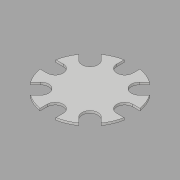
# Autodesk Inventor part: turntable
Saved by Autodesk Inventor 2017 (Build 210142000, 142)
## iProperties
Created: 2019-05-09
Part Number: turntable
Material: Generic
Document SubType Name: Modeling
Designer: Joe Sedutto
Density: 1 g/cm^3
Appearance: Default
Author: Joe Sedutto
Autodesk Inventor part; units mm, degrees
ref_plane "YZ Plane" through (0, 0, 0) normal (1, 0, 0) x (0, 1, 0)
ref_plane "XZ Plane" through (0, 0, 0) normal (0, 1, 0) x (-1, 0, 0)
ref_plane "XY Plane" through (0, 0, 0) normal (0, 0, 1) x (1, 0, 0)
sketch "Sketch1" plane through (0, 0, 0) normal (0, 1, 0) x (-1, 0, 0)
  circle A0 centre (0, 0) radius 34.925
  line L0 (0, 0) -> (0, -152.4) construction
  circle A1 centre (-107.7631, -44.6369) radius 34.925
  circle A2 centre (-152.4, -152.4) radius 34.925
  circle A3 centre (-107.7631, -260.1631) radius 34.925
  circle A4 centre (0, -304.8) radius 34.925
  circle A5 centre (107.7631, -260.1631) radius 34.925
  circle A6 centre (152.4, -152.4) radius 34.925
  circle A7 centre (107.7631, -44.6369) radius 34.925
  circle A8 centre (0, -152.4) radius 187.325
  dimension "d0" = 69.85
  dimension "d1" = 152.4
  dimension "d4" = 360
  constraints: 9 centre point, 2 coincident, 2 end point, 1 tangent, 1 vertical, 17 other
  measures "d0" diameter of A0
  measures "d1" distance of L0.end point (0, 0)
extrude "Extrusion1" add sketch "Sketch1" along normal blind 10
sketch "Sketch2" plane through (107.7631, 10, -44.6369) normal (0, 1, 0) x (1, 0, 0)
  arc A0 (-142.6881, -44.6369) -> (-72.8381, -44.6369) centre (-107.7631, -44.6369) ccw
  arc A1 (-142.6881, -76.2774) -> (-72.8381, -76.2774) centre (-107.7631, 107.7631) ccw
  line L0 (-72.8381, -44.6369) -> (-72.8381, -76.2774)
  line L1 (-142.6881, -44.6369) -> (-142.6881, -76.2774)
  circle A2 centre (-107.7631, -44.6369) radius 34.925 projected
  arc A3 (79.5619, 107.7631) -> (24.6957, 240.2219) centre (-107.7631, 107.7631) ccw projected
  arc A4 (-24.6957, -24.6957) -> (24.6957, 24.6957) centre (0, 0) ccw
  arc A5 (-2.3225, -47.0689) -> (47.0689, 2.3225) centre (-107.7631, 107.7631) ccw
  line L2 (24.6957, 24.6957) -> (47.0689, 2.3225)
  line L3 (-24.6957, -24.6957) -> (-2.3225, -47.0689)
  arc A6 (44.6369, 72.8381) -> (44.6369, 142.6881) centre (44.6369, 107.7631) ccw
  arc A7 (76.2774, 72.8381) -> (76.2774, 142.6881) centre (-107.7631, 107.7631) ccw
  line L4 (44.6369, 142.6881) -> (76.2774, 142.6881)
  line L5 (44.6369, 72.8381) -> (76.2774, 72.8381)
  arc A8 (24.6957, 190.8304) -> (-24.6957, 240.2219) centre (0, 215.5261) ccw
  arc A9 (47.0689, 213.2036) -> (-2.3225, 262.5951) centre (-107.7631, 107.7631) ccw
  line L6 (-24.6957, 240.2219) -> (-2.3225, 262.5951)
  line L7 (24.6957, 190.8304) -> (47.0689, 213.2036)
  arc A10 (-72.8381, 260.1631) -> (-142.6881, 260.1631) centre (-107.7631, 260.1631) ccw
  arc A11 (-72.8381, 291.8036) -> (-142.6881, 291.8036) centre (-107.7631, 107.7631) ccw
  line L8 (-142.6881, 260.1631) -> (-142.6881, 291.8036)
  line L9 (-72.8381, 260.1631) -> (-72.8381, 291.8036)
  arc A12 (-190.8304, 240.2219) -> (-240.2219, 190.8304) centre (-215.5261, 215.5261) ccw
  arc A13 (-213.2036, 262.5951) -> (-262.5951, 213.2036) centre (-107.7631, 107.7631) ccw
  line L10 (-240.2219, 190.8304) -> (-262.5951, 213.2036)
  line L11 (-190.8304, 240.2219) -> (-213.2036, 262.5951)
  arc A14 (-260.1631, 142.6881) -> (-260.1631, 72.8381) centre (-260.1631, 107.7631) ccw
  arc A15 (-291.8036, 142.6881) -> (-291.8036, 72.8381) centre (-107.7631, 107.7631) ccw
  line L12 (-260.1631, 72.8381) -> (-291.8036, 72.8381)
  line L13 (-260.1631, 142.6881) -> (-291.8036, 142.6881)
  arc A16 (-240.2219, 24.6957) -> (-190.8304, -24.6957) centre (-215.5261, 0) ccw
  arc A17 (-262.5951, 2.3225) -> (-213.2036, -47.0689) centre (-107.7631, 107.7631) ccw
  line L14 (-190.8304, -24.6957) -> (-213.2036, -47.0689)
  line L15 (-240.2219, 24.6957) -> (-262.5951, 2.3225)
  point P0 (-107.7631, -79.5619)
  point P1 (-107.7631, -79.5619)
  point P2 (24.6957, -24.6957)
  point P3 (79.5619, 107.7631)
  point P4 (24.6957, 240.2219)
  point P5 (-107.7631, 295.0881)
  point P6 (-240.2219, 240.2219)
  point P7 (-295.0881, 107.7631)
  point P8 (-240.2219, -24.6957)
  dimension "d10" = 360
  constraints: 42 point on circle, 32 end point, 16 centre point, 4 coincident, 2 tangent, 1 parallel, 1 vertical, 87 other
extrude "Extrusion2" cut sketch "Sketch2" against normal blind 10 contours A0 A1 L1 | A0 L0 A1 | A6 L4 A3 | A7 L5 A6 | L7 A8 A3 | A8 L6 A9 | A4 L2 A5 | A4 A5 L3 | A10 L8 A11 | A10 A11 L9 | A12 L10 A13 | A12 A13 L11 | A14 L12 A15 | A14 A15 L13 | A16 L14 A17 | A16 A17 L15
body "Solid1"
